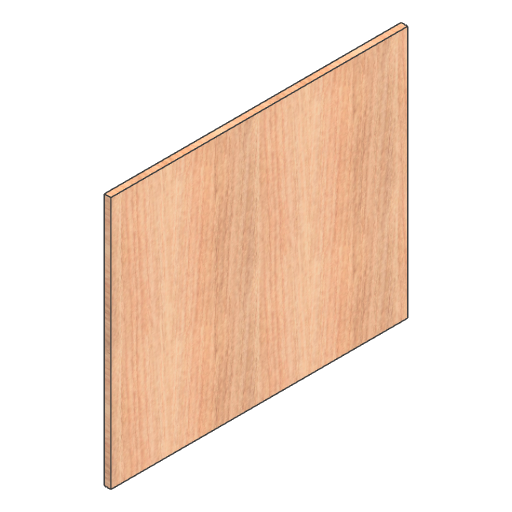
# Autodesk Inventor part: CUT PART J-01
Saved by Autodesk Inventor 2023.2 (Build 272271000, 271)
## iProperties
Created: 2022-11-02
Part Number: CUT PART J-01
Material: Wood (Birch)
Document SubType Name: Modeling
Designer: GUT
Density: 0.55 g/cm^3
Appearance: Birch - Natural Polished
Mass: 1669.01 g
Surface Area: 5299.76 cm^2
Volume: 3034.56 cm^3
d0: 464,000 mm
b: 545,000 mm
d2: 12,000 mm
d3: 0,00 deg
Author: GUT
Autodesk Inventor part; units mm, degrees
ref_plane "YZ Plane" through (0, 0, 0) normal (1, 0, 0) x (0, 1, 0)
ref_plane "XZ Plane" through (0, 0, 0) normal (0, 1, 0) x (-1, 0, 0)
ref_plane "XY Plane" through (0, 0, 0) normal (0, 0, 1) x (1, 0, 0)
sketch "Sketch1" plane through (0, 0, 0) normal (1, 0, 0) x (0, 1, 0)
  line L0 (-6.2078, -119.3085) -> (457.7922, -119.3085)
  line L1 (457.7922, -119.3085) -> (457.7922, -664.3085)
  line L2 (457.7922, -664.3085) -> (-6.2078, -664.3085)
  line L3 (-6.2078, -664.3085) -> (-6.2078, -119.3085)
  point P0 (0, 0)
  dimension "d0" = 464
  dimension "b" = 545
  constraints: 8 end point, 2 parallel, 1 horizontal, 1 perpendicular
  measures "d0" distance of L1.end L2.end
  measures "b" distance of L0.end L1.end
extrude "Extrusion1" add sketch "Sketch1" along normal blind 12
body "Solid1"
